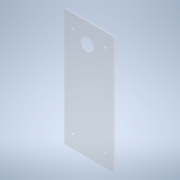
# Autodesk Inventor part: BaseC_4
Saved by Autodesk Inventor 2021 (Build 250183000, 183)
## iProperties
Created: 2023-10-20
Part Number: BaseC_4
Material: PMMA Plastic
Document SubType Name: Modeling
Designer: user
Density: 1.23963 g/cm^3
Appearance: Polycarbonate - Clear
Mass: 49.5 g
Surface Area: 285.037 cm^2
Volume: 39.9313 cm^3
Author: user
Autodesk Inventor part; units mm, degrees
ref_plane "YZ Plane" through (0, 0, 0) normal (1, 0, 0) x (0, 1, 0)
ref_plane "XZ Plane" through (0, 0, 0) normal (0, 1, 0) x (-1, 0, 0)
ref_plane "XY Plane" through (0, 0, 0) normal (0, 0, 1) x (1, 0, 0)
sketch "Sketch1" plane through (0, 0, 0) normal (0, 0, 1) x (1, 0, 0)
  line L0 (76, 0) -> (76, 180)
  line L1 (0, 180) -> (0, 0)
  line L2 (76, 180) -> (0, 180)
  circle A0 centre (35, 150) radius 10
  line L3 (0, 0) -> (76, 0)
  line L4 (13, 169.7925) -> (13, 8.2181)
  line L5 (63, 169.7925) -> (63, 4.1511)
  circle A1 centre (13, 160) radius 2.1
  circle A2 centre (63, 160) radius 2.1
  circle A3 centre (13, 20) radius 2.1
  circle A4 centre (63, 20) radius 2.1
  point P0 (63, 22.1)
  point P1 (63, 17.9)
  point P2 (13, 22.1)
  point P3 (13, 17.9)
  point P4 (63, 162.1)
  point P5 (63, 157.9)
  point P6 (13, 162.1)
  point P7 (13, 157.9)
  dimension "d1" = 180
  dimension "d26" = 20
  dimension "d27" = 35
  dimension "d28" = 30
  dimension "d29" = 180
  dimension "d30" = 13
  dimension "d31" = 13
  dimension "d32" = 4.2
  dimension "d33" = 4.2
  dimension "d34" = 20
  dimension "d35" = 20
  dimension "d36" = 4.2
  dimension "d37" = 4.2
  dimension "d38" = 20
  dimension "d39" = 20
  dimension "d40" = 76
  constraints: 12 end point, 5 centre point, 4 point on line, 2 vertical, 1 horizontal, 1 parallel
  measures "d1" distance of L0.end L0.start
  measures "d26" diameter of A0
  measures "d27" distance from line of L1 A0.centre
  measures "d28" distance from line of A0.centre L2
  measures "d29" distance of L1.start L1.end
  measures "d30" distance between parallel lines of L1 L4
  measures "d31" distance between parallel lines of L5 L0
  measures "d32" diameter of A1
  measures "d33" diameter of A2
  measures "d34" distance from line of A1.centre L2
  measures "d35" distance from line of A2.centre L2
  measures "d36" diameter of A3
  measures "d37" diameter of A4
  measures "d38" distance from line of L3 A4.centre
  measures "d39" distance from line of A3.centre L3
  measures "d40" distance between parallel lines of L1 L0
extrude "Extrusion1" add sketch "Sketch1" along normal blind 3
equation "\"d27\" = 0.5 * d0"
equation "\"d31\" = d30"
equation "\"d33\" = d32"
equation "\"d35\" = d34"
equation "\"d36\" = d33"
equation "\"d37\" = d36"
equation "\"d38\" = d39"
equation "\"d0\" = 70"
body "Solid1"
